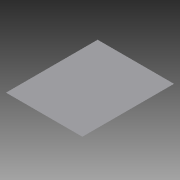
# Autodesk Inventor part: Wand1
Saved by Autodesk Inventor 2018.2 (Build 222227000, 227)
## iProperties
Created: 2019-02-06
Part Number: Wand1
Material: Generisch
Document SubType Name: Modeling
Designer: Lolob
Density: 1 g/cm^3
Appearance: Vorgabe
Author: Lolob
Autodesk Inventor part; units mm, degrees
ref_plane "YZ Plane" through (0, 0, 0) normal (1, 0, 0) x (0, 1, 0)
ref_plane "XZ Plane" through (0, 0, 0) normal (0, 1, 0) x (-1, 0, 0)
ref_plane "XY Plane" through (0, 0, 0) normal (0, 0, 1) x (1, 0, 0)
sketch "Skizze1" plane through (0, 0, 0) normal (0, 0, 1) x (1, 0, 0)
  line L0 (0, -420) -> (0, 420) projected
  line L1 (-350, 0) -> (350, 0) projected
  line L2 (-250, 300) -> (250, 300)
  line L3 (250, 300) -> (250, -300)
  line L4 (250, -300) -> (-250, -300)
  line L5 (-250, -300) -> (-250, 300)
  point P0 (0, 0)
  dimension "d0" = 500
  dimension "d1" = 600
  constraints: 8 end point, 2 parallel, 1 horizontal, 1 perpendicular, 2 other
  measures "d0" distance of L3.end L4.end
  measures "d1" distance of L4.end L2.start
extrude "Extrusion1" add sketch "Skizze1" along normal blind 20
chamfer "Fase1" distance 20 angle 45 4 edges at (-250, 0, 0) (0, 300, 0) (250, 0, 0) (0, -300, 0)
